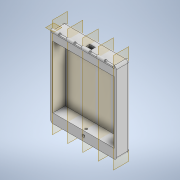
# Autodesk Inventor part: Bottom
Saved by Autodesk Inventor 2022 (Build 260153000, 153)
## iProperties
Created: 2022-03-05
Part Number: Bottom
Material: Generic
Document SubType Name: Modeling
Designer: Stump
Density: 1 g/cm^3
Appearance: Default
Author: Stump
Autodesk Inventor part; units mm, degrees
ref_plane "XZ Plane" through (0, 0, 0) normal (0, 1, 0) x (-1, 0, 0)
ref_plane "XY Plane" through (0, 0, 0) normal (0, 0, 1) x (1, 0, 0)
sketch "Sketch1" plane through (0, 0, 0) normal (0, 0, 1) x (1, 0, 0)
  line L0 (0, 0) -> (165.2524, 0)
  line L1 (165.2524, 0) -> (165.2524, 167.64)
  line L2 (165.2524, 167.64) -> (0, 167.64)
  line L3 (0, 167.64) -> (0, 0)
  line L4 (82.6262, 167.64) -> (82.6262, 193.04) construction
  line L5 (82.6262, 0) -> (82.6262, -25.4) construction
  line L6 (0, 83.82) -> (-6.35, 83.82) construction
  line L7 (165.2524, 83.82) -> (171.6024, 83.82) construction
  line L8 (-6.4155, -25.2979) -> (171.5352, -25.2979)
  line L9 (171.5352, -25.2979) -> (171.5352, 193.1152)
  line L10 (171.5352, 193.1152) -> (-6.4155, 193.1152)
  line L11 (-6.4155, 193.1152) -> (-6.4155, -25.2979)
  dimension "d0" = 165.2524
  dimension "d2" = 25.4
  dimension "d3" = 25.4
  dimension "d4" = 6.35
  dimension "d5" = 6.35
  constraints: 24 end point, 4 horizontal, 4 midpoint, 4 parallel, 2 perpendicular, 2 vertical
  measures "d0" distance of L2.end L1.end
  measures "d2" distance of L4.start L4.end
  measures "d3" distance of L5.start L5.end
  measures "d4" distance of L6.start L6.end
  measures "d5" distance of L7.start L7.end
extrude "Extrusion1" add sketch "Sketch1" along normal blind 37.592
sketch "Sketch3" plane through (0, 0, 0) normal (0, 0, -1) x (-1, 0, 0)
  line L0 (6.0775, -8.2655) -> (-172.3593, -8.2655)
  line L1 (-172.3593, -8.2655) -> (-172.3593, 173.0886)
  line L2 (-172.3593, 173.0886) -> (6.0775, 173.0886)
  line L3 (6.0775, 173.0886) -> (6.0775, -8.2655)
  point P0 (0, 0)
  constraints: 8 end point, 2 parallel, 1 horizontal, 1 perpendicular
extrude "Extrusion3" add sketch "Sketch3" against normal blind 4.699
fillet "Fillet1" radius 6.35 9 edges at (-6.4155, 193.1152, 18.796) (-6.4155, -25.2979, 18.796) (171.5352, -25.2979, 18.796) (171.5352, 193.1152, 18.796) (171.5352, -16.7817, 0) (171.5352, 183.1019, 0) (82.5599, -25.2979, 0) (-6.4155, 83.9087, 0) (82.5599, 193.1152, 0)
ref_plane "Work Plane1" through (0.254, 0, 0) normal (1, 0, 0) x (0, 1, 0)
ref_plane "Work Plane5" through (153.416, 0, 0) normal (1, 0, 0) x (0, 1, 0)
ref_plane "Work Plane6" through (0.254, 198.7479, 35.6964) normal (0, 1, 0) x (1, 0, 0)
sketch "Sketch10" plane through (0.254, 198.7479, 35.6964) normal (0, 1, 0) x (1, 0, 0)
  line L0 (0, -3.8053) -> (178.562, -3.8053) projected
  line L1 (178.562, 0) -> (178.562, -3.8053) projected
  line L2 (0, 0) -> (178.562, 0) projected
  line L3 (0, 0) -> (178.562, 0) projected
  line L4 (0, -7.6106) -> (178.562, -7.6106) projected
  line L5 (153.162, 0) -> (127.508, 0)
  line L6 (127.508, 0) -> (127.508, -7.6106)
  line L7 (127.508, -7.6106) -> (153.162, -7.6106)
  line L8 (153.162, -7.6106) -> (153.162, 0)
  line L9 (0, -7.6106) -> (178.562, -7.6106) projected
  line L10 (102.108, 0) -> (76.454, 0)
  line L11 (76.454, 0) -> (76.454, -7.6106)
  line L12 (76.454, -7.6106) -> (102.108, -7.6106)
  line L13 (102.108, -7.6106) -> (102.108, 0)
  line L14 (51.054, 0) -> (25.4, 0)
  line L15 (25.4, 0) -> (25.4, -7.6106)
  line L16 (25.4, -7.6106) -> (51.054, -7.6106)
  line L17 (51.054, -7.6106) -> (51.054, 0)
  line L18 (0, 0) -> (0, -3.8053) projected
  point P0 (-0.254, 35.6964)
  point P1 (25.4, 0)
  point P2 (51.054, -7.6106)
  point P3 (76.454, 0)
  constraints: 24 end point, 6 parallel, 5 point on line, 3 horizontal, 3 perpendicular
extrude "Extrusion9" cut sketch "Sketch10" against normal blind 5.715 contours L11 L2 L13 L0 | L0 L13 L4 L11 | L6 L2 L8 L0 | L0 L8 L4 L6
sketch "Sketch11" plane through (0, 0, 37.592) normal (0, 0, 1) x (1, 0, 0)
  line L0 (0, 0) -> (0, 167.64) projected
  line L1 (165.2524, 0) -> (0, 0) projected
  line L2 (165.2524, 167.64) -> (165.2524, 0) projected
  line L3 (0, 167.64) -> (165.2524, 167.64) projected
  line L4 (0, 0) -> (0, 167.64) projected
  line L5 (165.2524, 0) -> (0, 0) construction
  line L6 (82.6262, 0) -> (82.5599, -25.2979) construction
  line L7 (-0.0655, -25.2979) -> (165.1852, -25.2979) construction
  circle A0 centre (82.593, -12.6489) radius 3.7719
  dimension "d47" = 7.5438
  constraints: 3 midpoint, 2 end point, 1 centre point
  measures "d47" diameter of A0
extrude "Extrusion10" cut sketch "Sketch11" against normal blind 101.6 contours A0
sketch "Sketch13" plane through (0, 0, 0) normal (0, 0, -1) x (-1, 0, 0)
  circle A0 centre (-82.593, -12.6489) radius 3.7719 projected
  circle A1 centre (-82.593, -12.6489) radius 4.0259
  point P0 (0, 0)
  dimension "d50" = 8.0518
  constraints: 1 centre point, 1 coincident
  measures "d50" diameter of A1
extrude "Extrusion11" cut sketch "Sketch13" against normal blind 33.3502
sketch "Sketch14" plane through (0, 0, 37.592) normal (0, 1, 0) x (1, 0, 0)
  line L0 (86.3649, 4.2418) -> (78.8211, 4.2418) projected
  line L1 (82.593, 4.2418) -> (82.593, 10.5918)
  circle A0 centre (82.593, 7.4168) radius 3.1152
  point P0 (0, 37.592)
  dimension "d53" = 6.35
  constraints: 2 end point, 2 midpoint, 1 centre point, 1 vertical
  measures "d53" distance of L1.start L1.end
extrude "Extrusion12" cut sketch "Sketch14" against normal blind 19.05
sketch "Sketch17" plane through (0, 167.64, 37.592) normal (0, -1, 0) x (1, 0, 0)
  line L0 (165.1852, 0) -> (153.416, 0) projected
  line L1 (165.1852, -31.242) -> (165.1852, 0) projected
  line L2 (-0.0655, -31.242) -> (165.1852, -31.242) projected
  line L3 (-0.0655, 0) -> (-0.0655, -31.242) projected
  line L4 (-0.0655, -31.242) -> (165.1852, -31.242) projected
  line L5 (89.535, -31.242) -> (89.535, -17.5006)
  line L6 (89.535, -17.5006) -> (82.0801, -17.5006)
  line L7 (82.0801, -17.5006) -> (82.0801, -7.0104)
  line L8 (82.0801, -7.0104) -> (97.3201, -7.0104)
  line L9 (97.3201, -7.0104) -> (97.3201, -17.5006)
  line L10 (97.3201, -17.5006) -> (82.0801, -17.5006)
  line L11 (82.0801, -17.5006) -> (82.0801, -7.0104)
  line L12 (102.362, -1.8956) -> (102.362, 0) projected
  line L13 (127.762, 0) -> (102.362, 0) projected
  line L14 (127.762, 0) -> (127.762, -1.8956) projected
  line L15 (127.762, -1.8956) -> (153.416, -1.8956) projected
  line L16 (153.416, -1.8956) -> (153.416, 0) projected
  line L17 (76.708, 0) -> (-0.0655, 0) projected
  line L18 (76.708, 0) -> (76.708, -1.8956) projected
  line L19 (76.708, -1.8956) -> (102.362, -1.8956) projected
  point P0 (0, -37.592)
  dimension "d63" = 13.7414
  dimension "d64" = 7.4549
  dimension "d65" = 10.4902
  dimension "d66" = 15.24
  constraints: 14 end point, 3 perpendicular, 2 parallel, 1 horizontal, 1 point on line
  measures "d63" distance of L5.start L5.end
  measures "d64" distance of L5.end L6.end
  measures "d65" distance of L6.end L7.end
  measures "d66" distance of L9.end L10.end
extrude "Extrusion14" cut sketch "Sketch17" against normal blind 76.2 contours L6 L7 L8 L9 L10
sketch "Sketch18" plane through (0, 0, 0) normal (0, 0, -1) x (-1, 0, 0)
  circle A0 centre (-82.593, -12.6489) radius 3.7719 projected
  circle A1 centre (-82.593, -12.6489) radius 6.35
  point P0 (0, 0)
  dimension "d69" = 12.7
  constraints: 1 centre point, 1 coincident
  measures "d69" diameter of A1
extrude "Extrusion15" add sketch "Sketch18" against normal blind 2.54 contours A0 | A1
ref_plane "Work Plane7" through (165.354, 0, 0) normal (1, 0, 0) x (0, 1, 0)
sketch "Sketch19" plane through (0.254, 0, 0) normal (1, 0, 0) x (0, 1, 0)
  line L0 (186.7652, 37.592) -> (193.1152, 37.592) construction
  line L1 (193.1152, 37.592) -> (199.4652, 37.592) construction
  line L2 (199.4652, 37.592) -> (199.4652, 43.942) construction
  circle A0 centre (196.2902, 40.767) radius 3.175
  circle A1 centre (196.2902, 40.767) radius 1.5875
  point P0 (0, 0)
  dimension "d73" = 6.35
  dimension "d74" = 6.35
  dimension "d75" = 3.175
  constraints: 4 end point, 2 centre point, 1 coincident, 1 horizontal, 1 perpendicular
  measures "d73" distance of L0.end L1.end
  measures "d74" distance of L1.end L2.end
  measures "d75" diameter of A1
extrude "Extrusion16" add sketch "Sketch19" along normal blind 20.6375
sketch "Sketch20" plane through (0.254, 0, 0) normal (1, 0, 0) x (0, 1, 0)
  line L0 (194.2901, 40.767) -> (186.6701, 40.767)
  line L1 (186.6701, 40.767) -> (186.6701, 35.687)
  line L2 (186.6701, 35.687) -> (194.2901, 35.687)
  line L3 (194.2901, 38.9108) -> (194.2901, 40.767)
  line L4 (186.6701, 35.687) -> (196.2946, 35.687)
  line L5 (196.2946, 35.687) -> (196.2946, 38.9108)
  line L6 (196.2946, 38.9108) -> (194.2901, 38.9108)
  line L7 (186.6701, 38.9108) -> (186.6701, 35.687)
  point P0 (0, 0)
  dimension "d78" = 7.62
  dimension "d79" = 5.08
  constraints: 16 end point, 4 parallel, 2 horizontal, 2 perpendicular
  measures "d78" distance of L2.end L1.end
  measures "d79" distance of L1.end L0.end
extrude "Extrusion17" add sketch "Sketch20" along normal blind 165.1
ref_plane "Work Plane11" through (124.079, 0, 0) normal (1, 0, 0) x (0, 1, 0)
ref_plane "Work Plane10" through (82.804, 0, 0) normal (1, 0, 0) x (0, 1, 0)
sketch "Sketch23" plane through (41.529, 0, 0) normal (1, 0, 0) x (0, 1, 0)
  line L0 (193.113, 37.592) -> (186.6701, 37.592) projected
  line L1 (193.113, 37.592) -> (199.463, 37.592)
  line L2 (199.463, 37.592) -> (199.463, 43.942)
  circle A0 centre (196.288, 40.767) radius 3.175
  circle A1 centre (196.288, 40.767) radius 1.5875
  point P0 (0, 0)
  dimension "d96" = 6.35
  dimension "d97" = 6.35
  dimension "d98" = 3.175
  constraints: 4 end point, 2 centre point, 1 coincident, 1 horizontal, 1 perpendicular
  measures "d96" distance of L0.start L1.end
  measures "d97" distance of L1.end L2.end
  measures "d98" diameter of A1
extrude "Extrusion20" add sketch "Sketch23" along normal blind 20.6375 contours A0
sketch "Sketch24" plane through (82.804, 0, 0) normal (1, 0, 0) x (0, 1, 0)
  line L0 (193.113, 35.687) -> (193.113, 37.592) projected
  line L1 (193.113, 37.592) -> (199.463, 37.592)
  line L2 (199.463, 37.592) -> (199.463, 43.942)
  circle A0 centre (196.288, 40.767) radius 3.175
  circle A1 centre (196.288, 40.767) radius 1.5875
  point P0 (0, 0)
  dimension "d101" = 6.35
  dimension "d102" = 6.35
  dimension "d103" = 3.175
  constraints: 4 end point, 2 centre point, 1 coincident, 1 horizontal, 1 perpendicular
  measures "d101" distance of L0.end L1.end
  measures "d102" distance of L1.end L2.end
  measures "d103" diameter of A1
extrude "Extrusion21" add sketch "Sketch24" along normal blind 20.6375 contours A0
sketch "Sketch25" plane through (124.079, 0, 0) normal (1, 0, 0) x (0, 1, 0)
  line L0 (193.113, 37.592) -> (186.6701, 37.592) projected
  line L1 (193.113, 37.592) -> (199.463, 37.592)
  line L2 (199.463, 37.592) -> (199.463, 43.942)
  circle A0 centre (196.288, 40.767) radius 3.175
  circle A1 centre (196.288, 40.767) radius 1.5875
  point P0 (0, 0)
  dimension "d106" = 6.35
  dimension "d107" = 6.35
  dimension "d108" = 3.175
  constraints: 4 end point, 2 centre point, 1 coincident, 1 horizontal, 1 perpendicular
  measures "d106" distance of L0.start L1.end
  measures "d107" distance of L1.end L2.end
  measures "d108" diameter of A1
extrude "Extrusion22" add sketch "Sketch25" along normal blind 20.6375 contours A0
fillet "Fillet4" radius 3.175 1 edges at (82.804, 186.6701, 40.767)
sketch "Sketch26" plane through (0.254, 196.2946, 35.687) normal (0, 1, 0) x (1, 0, 0)
  line L0 (144.4625, -1.905) -> (144.4625, -3.2238) projected
  line L1 (144.4625, -3.2238) -> (165.1, -3.2238) projected
  line L2 (165.1, 0) -> (165.1, -3.2238) projected
  line L3 (0, 0) -> (165.1, 0) projected
  line L4 (0, 0) -> (0, -1.905) projected
  line L5 (20.6375, -1.905) -> (0, -1.905) projected
  line L6 (20.6375, -3.2238) -> (20.6375, -1.905) projected
  line L7 (20.6375, -3.2238) -> (41.275, -3.2238) projected
  line L8 (41.275, -3.2238) -> (41.275, -1.905) projected
  line L9 (41.275, -1.905) -> (61.9125, -1.905) projected
  line L10 (61.9125, -1.905) -> (61.9125, -3.2238) projected
  line L11 (61.9125, -3.2238) -> (82.55, -3.2238) projected
  line L12 (82.55, -3.2238) -> (82.55, -1.905) projected
  line L13 (82.55, -1.905) -> (103.1875, -1.905) projected
  line L14 (103.1875, -1.905) -> (103.1875, -3.2238) projected
  line L15 (103.1875, -3.2238) -> (123.825, -3.2238) projected
  line L16 (123.825, -3.2238) -> (123.825, -1.905) projected
  line L17 (123.825, -1.905) -> (144.4625, -1.905) projected
  line L18 (123.825, -8.255) -> (144.4625, -8.255) projected
  line L19 (165.1, 0) -> (144.4625, 0)
  line L20 (144.4625, 0) -> (144.4625, -8.255)
  line L21 (144.4625, -8.255) -> (165.1, -8.255)
  line L22 (165.1, -8.255) -> (165.1, 0)
  line L23 (0, 0) -> (165.1, 0) projected
  line L24 (123.825, 0) -> (103.1875, 0)
  line L25 (103.1875, 0) -> (103.1875, -8.255)
  line L26 (103.1875, -8.255) -> (123.825, -8.255)
  line L27 (123.825, -8.255) -> (123.825, 0)
  line L28 (82.55, 0) -> (61.9125, 0)
  line L29 (61.9125, 0) -> (61.9125, -8.255)
  line L30 (61.9125, -8.255) -> (82.55, -8.255)
  line L31 (82.55, -8.255) -> (82.55, 0)
  line L32 (41.275, 0) -> (20.6375, 0)
  line L33 (20.6375, 0) -> (20.6375, -8.255)
  line L34 (20.6375, -8.255) -> (41.275, -8.255)
  line L35 (41.275, -8.255) -> (41.275, 0)
  point P0 (-0.254, 35.687)
  point P1 (20.6375, 0)
  point P2 (61.9125, 0)
  constraints: 32 end point, 8 parallel, 6 point on line, 4 horizontal, 4 perpendicular, 1 midpoint
extrude "Extrusion23" cut sketch "Sketch26" against normal blind 3.175 contours L20 L3 L2 L1 L0 | L1 L22 L21 L20 | L16 L15 L14 L25 L3 L27 | L27 L26 L25 L15 | L31 L12 L11 L10 L29 L3 | L31 L30 L29 L11 | L35 L8 L7 L6 L33 L3 | L35 L34 L33 L7
fillet "Fillet5" radius 3.175 4 edges at (10.5728, 196.2946, 35.687) (51.8477, 196.2946, 35.687) (93.1228, 196.2946, 35.687) (134.3978, 196.2946, 35.687)
ref_plane "Work Plane9" through (41.529, 0, 0) normal (1, 0, 0) x (0, 1, 0)
body "Solid1"
